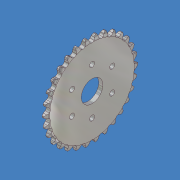
# Autodesk Inventor part: AM-0146 S35-30 Sprocket
Saved by Autodesk Inventor 2013 (Build 170138000, 138)
## iProperties
Category: iParts
Company: FirstCadLibrary
Shininess: 64.0
Length Units: 11272
Angle Units: 11279
Time Units: 11290
Mass Units: 11286
Length Display Precision: 3
Angle Display Precision: 2
Compacted: True
Part Number: AM-0146 S35-30 Sprocket
Document SubType Name: Modeling
Created: 2006-02-06
Designer: Ed Sparks
Material: Aluminum-6061
Engineer: Ed Sparks
Density: 7.86 g/cm^3
Density: 0.0
Volumn: 0.0
Area: 0.0
PropertySet Name: Model Information
Control State: 0
Master: False
Checked Out: False
Title: i-Sprocket
Subject: i-Sprocket
Author: Ed Sparks
Keywords: Sprocket
Autodesk Inventor part; units mm, degrees
ref_plane "YZ Plane" through (0, 0, 0) normal (1, 0, 0) x (0, 1, 0)
ref_plane "XZ Plane" through (0, 0, 0) normal (0, 1, 0) x (-1, 0, 0)
ref_plane "XY Plane" through (0, 0, 0) normal (0, 0, 1) x (1, 0, 0)
sketch "Sketch1" plane through (0, 0, 0) normal (0, 0, 1) x (1, 0, 0)
  line L0 (-2.1384, 0) -> (2.1384, 0)
  line L1 (0, 0) -> (0, 48.1697) construction
  line L2 (-0.9484, 48.1697) -> (0.9484, 48.1697)
  line L3 (-2.1384, 0) -> (-2.1384, 43.4072)
  line L4 (2.1384, 0) -> (2.1384, 43.4072)
  arc A0 (-0.9484, 48.1697) -> (-2.1384, 43.4072) centre (7.9867, 43.4072) ccw
  arc A1 (2.1384, 43.4072) -> (0.9484, 48.1697) centre (-7.9867, 43.4072) ccw
  point P0 (25.317, 18.8926)
  dimension "d0" = 4.2767
  dimension "d1" = 48.1697
  dimension "d2" = 4.7625
  dimension "d3" = 10.1251
  constraints: 10 end point, 4 point on circle, 2 centre point, 2 coincident, 2 horizontal, 2 horizontal alignment, 2 midpoint, 2 parallel, 2 perpendicular, 2 symmetric about line, 1 other
  measures "d0" distance of L0.start L0.end
  measures "d1" distance between parallel lines of L0 L2
  measures "d2" distance from line of point (7.987, 43.407) L2
  measures "d3" distance of point (7.987, 43.407) L3.end
revolve "Sprocket Blank" add sketch "Sketch1" angle 360 about axis through (-2.1384, 0, 0) along (1, 0, 0)
sketch "Sketch2" plane through (2.1384, 0, 0) normal (1, 0, 0) x (0, 0, -1)
  circle A0 centre (0, 0) radius 43.4072 projected
  line L0 (0, 0) -> (0, 35.1967) construction
  circle A1 centre (0, 0) radius 45.5618 construction
  line L1 (0, 0) -> (3.7817, 35.9805) construction
  arc A2 (-2.0691, 44.0026) -> (2.0691, 44.0026) centre (0, 45.5618) ccw
  arc A3 (2.0691, 44.0026) -> (3.1106, 46.0366) centre (-3.2457, 48.0075) ccw
  arc A4 (-3.1106, 46.0366) -> (-2.0691, 44.0026) centre (3.2457, 48.0075) ccw
  line L2 (0, 0) -> (-3.6485, 34.7128) construction
  arc A5 (-3.1106, 46.0366) -> (-5.0907, 48.4351) centre (-7.0225, 44.8237) ccw
  arc A6 (5.0907, 48.4351) -> (3.1106, 46.0366) centre (7.0225, 44.8237) ccw
  arc A7 (5.0907, 48.4351) -> (-5.0907, 48.4351) centre (0, 0) ccw
  dimension "d9" = 91.1235
  dimension "d10" = 6
  dimension "d11" = 7.0225
  dimension "d12" = 3.2456
  dimension "d13" = 0.7381
  dimension "d15" = 2.4458
  dimension "d17" = 5.1816
  constraints: 14 coincident, 12 point on circle, 6 centre point, 6 end point, 3 point on line, 3 tangent, 2 horizontal alignment, 2 symmetric about line, 1 vertical, 1 vertical alignment, 5 other
  measures "d10" angle of L1 L0
  measures "d11" horizontal distance of point (7.023, 44.824) L0.start
  measures "d12" horizontal distance of point (-3.246, 48.008) L0.start
  measures "d13" vertical distance of point (7.023, 44.824) point (0, 45.562)
  measures "d15" vertical distance of point (0, 45.562) point (-3.246, 48.008)
  measures "d17" diameter of A2
extrude "Tooth Profile" cut sketch "Sketch2" against normal blind 25.4 contours A2 A0 | A0 A2 A4 A5 A7 A6 A3 picked at (-0.0987, 43.2658)
sketch "Sketch5" plane through (-2.1384, 0, 0) normal (-1, 0, 0) x (0, 0, 1)
  circle A0 centre (0, 0) radius 43.4072 projected
  constraints: 1 coincident
hole "Bore" at (-2.1384, 0, 0) direction (1, 0, 0) diameter 22.2123 end through all
pattern_circular "Circular Pattern2" count 30 over 360 about axis through (-10, 0, 0) along (1, 0, 0) of "Tooth Profile"
sketch "Sketch10" plane through (2.1384, 45.5618, 0) normal (1, 0, 0) x (0, 0, -1)
  arc A0 (41.695, -57.6329) -> (1.4041, -2.1773) centre (0, -45.5618) ccw projected
  line L0 (0, -45.5618) -> (0, -0.9271) construction
  point P0 (0, -21.7493)
  dimension "d56" = 23.8125
  constraints: 2 end point, 1 coincident, 1 point on line, 1 vertical
  measures "d56" distance of point (0, -21.749) A0.centre
hole "Hole3" at (2.1384, 23.8125, 0) direction (-1, 0, 0) diameter 5.2324 end through all
pattern_circular "Circular Pattern3" count 6 over 360 about axis through (134.031, 0, 0) along (-1, 0, 0) of "Hole3"
equation "\"d0\" = Sprocket_Thickness"
equation "\"d1\" = Outside_Radius"
equation "\"d2\" = Depth_Of_Chamfer"
equation "\"d3\" = Chamfer_Radius"
equation "\"d9\" = Pitch_Diameter"
equation "\"d11\" = W_"
equation "\"d12\" = M_"
equation "\"d13\" = V_"
equation "\"d15\" = T_"
equation "\"d17\" = Seating_Curve_Diameter"
equation "\"d42\" = Bore_Diameter"
equation "\"Chamfer_Radius\" = 1.063 * Chain_Pitch"
equation "\"Depth_Of_Chamfer\" = 0.5 * Chain_Pitch"
equation "\"Chain_Pitch\" = 9.525"
equation "\"Roller_Diameter\" = 5.08"
equation "\"d14\" = F_"
equation "\"d16\" = E_"
equation "\"Hub_Diameter\" = 37.30625"
equation "\"Bore_Diameter\" = 22.2123"
equation "\"Length_Through_Bore\" = 19.05"
equation "\"Key_Width\" = 3.175"
equation "\"Hub_Chamfer\" = 0.254"
equation "\"Sprocket_Thickness\" = 4.276725"
equation "\"Outside_Radius\" = 48.169661"
equation "\"Pitch_Diameter\" = 91.123506"
equation "\"Seating_Curve_Diameter\" = 5.1816"
equation "\"F_\" = 4.12308"
equation "\"E_\" = 6.6548"
equation "\"W_\" = 7.022518"
equation "\"M_\" = 3.245655"
equation "\"V_\" = 0.738096"
equation "\"T_\" = 2.445776"
body "Solid1"
